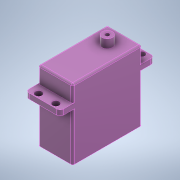
# Autodesk Inventor part: ServoMotor(20kg・cm)
Saved by Autodesk Inventor 2022 (Build 260153000, 153)
## iProperties
Created: 2024-09-20
Part Number: ServoMotor(20kg・cm)
Material: 一般
Document SubType Name: Modeling
Designer: acbaf
Density: 1 g/cm^3
Appearance: 滑らか - 紫
Author: acbaf
Autodesk Inventor part; units mm, degrees
sketch "スケッチ1" plane through (0, 0, 0) normal (0, 1, 0) x (-1, 0, 0)
  line L0 (0, 0) -> (-20, 0)
  line L1 (-20, 0) -> (-20, -40)
  line L2 (-20, -40) -> (0, -40)
  line L3 (0, -40) -> (0, 0)
  line L4 (0, -44.75) -> (-20, -44.75)
  line L5 (-20, -44.75) -> (-20, 4.75)
  line L6 (-20, 4.75) -> (0, 4.75)
  line L7 (0, 4.75) -> (0, -44.75)
  line L8 (-2, -47.25) -> (-18, -47.25)
  line L9 (-20, -45.25) -> (-20, 5.25)
  line L10 (-18, 7.25) -> (-2, 7.25)
  line L11 (0, 5.25) -> (0, -45.25)
  line L12 (-10, -61.4419) -> (-10, 22.3426)
  arc A0 (0, 5.25) -> (-2, 7.25) centre (-2, 5.25) ccw
  arc A1 (-18, 7.25) -> (-20, 5.25) centre (-18, 5.25) ccw
  arc A2 (-20, -45.25) -> (-18, -47.25) centre (-18, -45.25) ccw
  arc A3 (-2, -47.25) -> (0, -45.25) centre (-2, -45.25) ccw
  circle A4 centre (-10, -30) radius 3
  line L13 (-6.5, -45) -> (-13.5, -45)
  line L14 (-13.5, -45) -> (-13.5, -40)
  line L15 (-13.5, -40) -> (-6.5, -40)
  line L16 (-6.5, -40) -> (-6.5, -45)
  circle A5 centre (-10, -30) radius 1.25
  point P0 (-10, -20)
  point P1 (-20, 7.25)
  point P2 (-20, -47.25)
  point P3 (0, 7.25)
  point P4 (-5, 4.75)
  point P5 (-15, 4.75)
  point P6 (-20, 4.75)
  point P7 (-6.5, 0)
  point P8 (-13.5, 0)
  dimension "d0" = 20
  dimension "d1" = 40
  dimension "d2" = 20
  dimension "d3" = 49.5
  dimension "d4" = 20
  dimension "d5" = 54.5
  dimension "d6" = 24.75
  dimension "d7" = 27.25
  dimension "d8" = 10
  dimension "d9" = 0
  dimension "d10" = 0
  dimension "d11" = 4.75
  dimension "d12" = 0
  dimension "d13" = 10
  dimension "d14" = 10
  dimension "d15" = 5
  dimension "d16" = 2
  dimension "d30" = 6
  dimension "d33" = 7
  dimension "d34" = 5
  dimension "d35" = 3.5
  dimension "d42" = 2.5
  dimension "d45" = 0
  constraints: 34 end point, 9 point on line, 8 parallel, 8 point on circle, 8 tangent, 6 centre point, 4 horizontal, 4 perpendicular, 3 equal radius, 2 coincident, 1 vertical
  measures "d0" distance of L2.end L1.end
  measures "d1" distance of L1.end L0.end
  measures "d2" distance of L5.end L6.end
  measures "d3" distance of L4.end L5.end
  measures "d4" distance of point (-20, 7.25) point (0, 7.25)
  measures "d5" distance of point (-20, -47.25) point (-20, 7.25)
  measures "d6" distance from line of L4 point (-10, -20)
  measures "d7" distance from line of L8 point (-10, -20)
  measures "d8" distance from line of L1 point (-10, -20)
  measures "d9" distance between parallel lines of L7 L3
  measures "d10" distance between parallel lines of L11 L3
  measures "d11" distance between parallel lines of L4 L2
  measures "d12" distance from line of L12 point (-10, -20)
  measures "d13" distance from line of L2 point (-10, -30)
  measures "d14" distance of point (-15, 4.75) point (-5, 4.75)
  measures "d15" distance from line of L7 point (-5, 4.75)
  measures "d16" radius of A0
  measures "d30" diameter of A4
  measures "d33" distance of L14.end L15.end
  measures "d34" distance of L13.end L14.end
  measures "d35" distance between parallel lines of L12 L16
  measures "d42" diameter of A5
  measures "d45" distance between parallel lines of L2 L15
extrude "押し出し1" add sketch "スケッチ1" along normal blind 40.5 contours L3 L2 L12 A4 L0 | L12 A4 L2 L1 L0 | A4 L12 A5 | L12 A5 A4 | A5 L12 | L12 A5
ref_plane "作業平面1" through (0, 27.8, 0) normal (0, -1, 0) x (1, 0, 0)
extrude "押し出し2" add sketch "スケッチ1" along normal blind 3.1 from surface at 27.8 contours L0 L12 L6 L7 | L0 L5 L6 L12 | L7 L4 L16 L2 | L6 L12 L10 A0 L11 | L6 L9 A1 L10 L12 | L16 L4 L12 L2 | L11 A3 L8 L12 L13 L16 L4 | L2 L14 L4 L5 | L12 L4 L14 L2 | L16 L13 L12 L4 | L4 L14 L13 L12 L8 A2 L9 | L12 L13 L14 L4
hole "穴1" at (5, 0, 4.75) at (15, 0, 4.75) direction (0, 1, 0) diameter 4 end through all
ref_plane "作業平面2" through (0, 40.5, -20) normal (0, 0, 1) x (1, 0, 0)
mirror "ミラー1" about plane through (0, 40.5, -20) normal (0, 0, 1) of "穴1"
extrude "押し出し3" add sketch "スケッチ1" along normal blind 5 from surface at 40.5 contours A4 L12 A5 | L12 A5 A4 | A5 L12 | L12 A5
ref_plane "作業平面3" through (0, 8, 0) normal (0, -1, 0) x (1, 0, 0)
extrude "押し出し4" add sketch "スケッチ1" against normal blind 4 from surface at 8 contours L16 L4 L12 L2 | L12 L4 L14 L2 | L16 L13 L12 L4 | L12 L13 L14 L4
fillet "フィレット1" radius 1 12 edges at (0, 35.7, 0) (0, 13.9, 0) (20, 13.9, 0) (20, 35.7, 0) (20, 13.9, -40) (20, 35.7, -40) (0, 13.9, -40) (0, 35.7, -40) (20, 40.5, -20) (0, 40.5, -20) (10, 40.5, 0) (10, 40.5, -40)
extrude "押し出し5" cut sketch "スケッチ1" against normal blind 4 from surface at 45.5 contours A5 L12 | L12 A5
equation "\"d6\" = 0.5 * d3"
equation "\"d7\" = 0.5 * d5"
equation "\"d8\" = 0.5 * d2"
equation "\"d35\" = 0.5 * d33"
